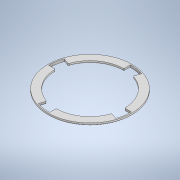
# Autodesk Inventor part: capLockBottom4
Saved by Autodesk Inventor 2020 (Build 240168000, 168)
## iProperties
Created: 2019-08-14
Part Number: capLockBottom4
Material: Generic
Document SubType Name: Modeling
Designer: alejandrosalazar
Density: 1 g/cm^3
Appearance: Default
Author: alejandrosalazar
Autodesk Inventor part; units mm, degrees
ref_plane "YZ Plane" through (0, 0, 0) normal (1, 0, 0) x (0, 1, 0)
ref_plane "XZ Plane" through (0, 0, 0) normal (0, 1, 0) x (-1, 0, 0)
ref_plane "XY Plane" through (0, 0, 0) normal (0, 0, 1) x (1, 0, 0)
sketch "Sketch1" plane through (0, 0, 0) normal (0, 1, 0) x (-1, 0, 0)
  circle A0 centre (0, 0) radius 35
  line L0 (0, 0) -> (34, 0) construction
  line L1 (-0.3543, 28.9978) -> (-0.4154, 33.9975)
  line L2 (0, 0) -> (34, 0) construction
  line L3 (9.1538, 27.5174) -> (10.7321, 32.2618)
  line L4 (0, 0) -> (34, 0) construction
  line L5 (28.9978, 0.3543) -> (33.9975, 0.4154)
  line L6 (0, 0) -> (34, 0) construction
  line L7 (27.5174, -9.1538) -> (32.2618, -10.7321)
  line L8 (0, 0) -> (34, 0) construction
  line L9 (0.3543, -28.9978) -> (0.4154, -33.9975)
  line L10 (0, 0) -> (34, 0) construction
  line L11 (-9.1538, -27.5174) -> (-10.7321, -32.2618)
  line L12 (0, 0) -> (34, 0) construction
  line L13 (-28.9978, -0.3543) -> (-33.9975, -0.4154)
  line L14 (0, 0) -> (34, 0) construction
  line L15 (-27.5174, 9.1538) -> (-32.2618, 10.7321)
  line L16 (0, 0) -> (34, 0) construction
  arc A1 (-0.3543, 28.9978) -> (-27.5174, 9.1538) centre (0, 0) ccw
  arc A2 (-32.2618, 10.7321) -> (-33.9975, -0.4154) centre (0, 0) ccw
  arc A3 (-28.9978, -0.3543) -> (-9.1538, -27.5174) centre (0, 0) ccw
  arc A4 (-10.7321, -32.2618) -> (0.4154, -33.9975) centre (0, 0) ccw
  arc A5 (0.3543, -28.9978) -> (27.5174, -9.1538) centre (0, 0) ccw
  arc A6 (29, 0) -> (9.1538, 27.5174) centre (0, 0) ccw
  arc A7 (32.2618, -10.7321) -> (33.9975, 0.4154) centre (0, 0) ccw
  arc A8 (10.7321, 32.2618) -> (-0.4154, 33.9975) centre (0, 0) ccw
  dimension "d0" = 70
  dimension "d4" = 90.7
  dimension "d5" = 71.6
  dimension "d6" = 0.7
  dimension "d7" = 18.4
  dimension "d8" = 89.3
  dimension "d9" = 108.4
  dimension "d10" = 179.3
  dimension "d11" = 161.6
  constraints: 34 end point, 17 point on circle, 9 centre point, 9 horizontal, 3 coincident, 1 point on line
  measures "d0" diameter of A0
  measures "d4" angle of L2 L1
  measures "d5" angle of L4 L3
  measures "d6" angle of L6 L5
  measures "d7" angle of L7 L8
  measures "d8" angle of L9 L10
  measures "d9" angle of L11 L12
  measures "d10" angle of L13 L14
  measures "d11" angle of L16 L15
extrude "Extrusion1" add sketch "Sketch1" along normal blind 2
fillet "Fillet7" radius 0.7 1 edges at (35, 0, 0)
sketch "Sketch5" plane through (0, 2, 0) normal (0, 1, 0) x (1, 0, 0)
  circle A0 centre (0, 0) radius 28.55
  line L0 (-32.2618, 10.7321) -> (-27.5174, 9.1538) projected
  line L1 (0, 0) -> (-27.5174, 9.1538)
  line L2 (28.9978, 0.3543) -> (33.9975, 0.4154) projected
  line L3 (28.9978, 0.3543) -> (-28.9978, -0.3543)
  arc A1 (-28.9978, -0.3543) -> (-9.1538, -27.5174) centre (0, 0) ccw projected
  arc A2 (28.9978, 0.3543) -> (9.1538, 27.5174) centre (0, 0) ccw projected
  line L4 (-10.7321, -32.2618) -> (-9.1538, -27.5174) projected
  line L5 (9.1538, 27.5174) -> (-9.1538, -27.5174)
  arc A3 (0.3543, -28.9978) -> (27.5174, -9.1538) centre (0, 0) ccw projected
  line L6 (0.3543, -28.9978) -> (-0.3543, 28.9978)
  line L7 (0.3543, -28.9978) -> (0.4154, -33.9975) projected
  line L8 (32.2618, -10.7321) -> (27.5174, -9.1538) projected
  line L9 (27.5174, -9.1538) -> (0, 0)
  circle A4 centre (0, 0) radius 29
  point P0 (-27.0904, 9.0118)
  point P1 (-0.3488, 28.5479)
  point P2 (9.0118, 27.0904)
  point P3 (28.5479, 0.3488)
  point P4 (27.0904, -9.0118)
  point P5 (0.3488, -28.5479)
  point P6 (-9.0118, -27.0904)
  point P7 (-28.5479, -0.3488)
  dimension "d53" = 57.1
  dimension "d54" = 58
  constraints: 10 end point, 4 collinear, 2 centre point, 2 coincident, 1 point on circle
  measures "d53" diameter of A0
  measures "d54" diameter of A4
extrude "Extrusion5" add sketch "Sketch5" against normal blind 2 contours A0 L5 A2 L3 | L9 A3 L6 A0 | A0 L1 A4 L6 | A0 L5 A1 L3
fillet "Fillet11" radius 0.7 4 edges at (-23.0534, 0, 16.8417) (-16.8417, 0, -23.0534) (23.0534, 0, -16.8417) (16.8417, 0, 23.0534)
fillet "Fillet12" radius 0.5 24 edges at (-0.3488, 1.35, -28.5479) (-0.3513, 0.205, -28.7529) (-0.3864, 0, -31.6226) (9.0118, 1.35, -27.0904) (9.0765, 0.205, -27.285) (9.9824, 0, -30.0082) (-28.5479, 1.35, 0.3488) (-28.7529, 0.205, 0.3513) (-31.6226, 0, 0.3864) (-27.0904, 1.35, -9.0118) (-27.285, 0.205, -9.0765) (-30.0082, 0, -9.9824) (-9.0118, 1.35, 27.0904) (-9.0765, 0.205, 27.285) (-9.9824, 0, 30.0082) (0.3488, 1.35, 28.5479) (0.3513, 0.205, 28.7529) (0.3864, 0, 31.6226) (27.0904, 1.35, 9.0118) (27.285, 0.205, 9.0765) (30.0082, 0, 9.9824) (28.5479, 1.35, -0.3488) (28.7529, 0.205, -0.3513) (31.6226, 0, -0.3864)
body "Solid1"
